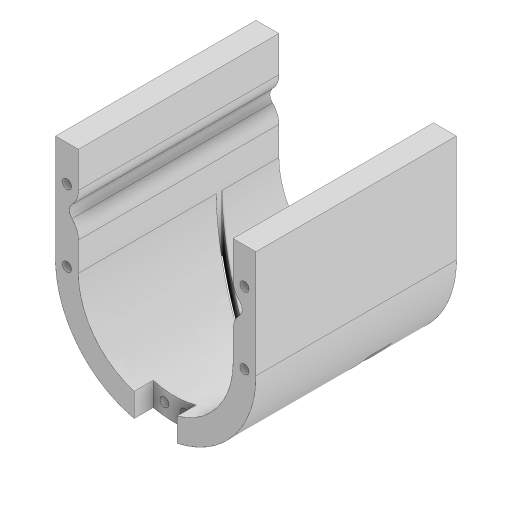
# Autodesk Inventor part: front wall
Saved by Autodesk Inventor 2024 (Build 280153000, 153)
## iProperties
Created: 2024-08-03
Part Number: front wall
Material: Generic
Document SubType Name: Modeling
Designer: chris
Density: 1 g/cm^3
Appearance: Default
Author: chris
Autodesk Inventor part; units mm, degrees
ref_plane "YZ Plane" through (0, 0, 0) normal (1, 0, 0) x (0, 1, 0)
ref_plane "XZ Plane" through (0, 0, 0) normal (0, 1, 0) x (-1, 0, 0)
ref_plane "XY Plane" through (0, 0, 0) normal (0, 0, 1) x (1, 0, 0)
sketch "Sketch1" plane through (0, 0, 0) normal (0, 0, 1) x (1, 0, 0)
  circle A0 centre (-39.37, 31.75) radius 2
  circle A1 centre (39.37, 31.75) radius 2
  circle A2 centre (39.37, 0) radius 2
  circle A3 centre (-39.37, 0) radius 2
  circle A4 centre (-4.5035, -38.773) radius 2
  circle A5 centre (4.4965, -38.773) radius 2
  arc A6 (-44.45, 0) -> (44.45, 0) centre (0, 0) ccw
  line L0 (44.45, 0) -> (44.45, 47.625)
  line L1 (-44.45, 47.625) -> (-44.45, 0)
  line L2 (-39.37, 47.625) -> (-44.45, 47.625)
  line L3 (-34.29, 37.465) -> (-34.29, 0)
  arc A7 (-34.29, 0) -> (34.29, 0) centre (0, 0) ccw
  line L4 (34.29, 0) -> (34.29, 37.465)
  line L5 (-34.29, 37.465) -> (-34.29, 47.625)
  line L6 (34.29, 37.465) -> (34.29, 47.625)
  line L7 (-39.37, 47.625) -> (-34.29, 47.625)
  line L8 (34.29, 47.625) -> (44.45, 47.625)
  circle A8 centre (198.4277, -79.2169) radius 2
  circle A9 centre (277.1677, -79.2169) radius 2
  circle A10 centre (277.1677, -110.9669) radius 2
  circle A11 centre (198.4277, -110.9669) radius 2
  circle A12 centre (233.2942, -149.74) radius 2
  circle A13 centre (242.2942, -149.74) radius 2
  arc A14 (193.3477, -110.9669) -> (282.2477, -110.9669) centre (237.7977, -110.9669) ccw
  line L9 (282.2477, -110.9669) -> (282.2477, 11.3384)
  line L10 (193.3477, 11.3384) -> (193.3477, -110.9669)
  line L11 (198.4277, -47.4669) -> (198.4277, -79.2169)
  line L12 (198.4277, -63.3419) -> (183.6023, -63.3419)
  line L13 (198.4277, -63.3419) -> (302.3131, -63.3419)
  circle A15 centre (-34.5, 22.2747) radius 2
  circle A16 centre (34.5, 22.2747) radius 2
  circle A17 centre (-34.5, 22.2747) radius 3.81
  circle A18 centre (34.5, 22.2747) radius 3.81
  point P0 (0, 0)
  point P1 (-0.0035, -24.273)
  point P2 (237.7942, -135.24)
  point P3 (-34.29, 26.0789)
  point P4 (-34.29, 18.4704)
  point P5 (34.29, 24.2636)
  point P6 (34.29, 20.2857)
  point P7 (34.29, 18.4704)
  point P8 (34.29, 26.0789)
  dimension "d8" = 7.62
  dimension "d9" = 7.62
  constraints: 28 end point, 19 centre point, 6 point on circle, 3 horizontal, 3 vertical, 2 coincident, 2 perpendicular, 1 midpoint, 2 other
  measures "d8" diameter of A17
  measures "d9" diameter of A18
extrude "Extrusion1" add sketch "Sketch1" along normal blind 88.9 contours A4 | A5 | L1 L2 L7 L5 L3 A17 A7 L4 A18 L6 L8 L0 A6 | A18 L4 A16 | L3 A15 A17 | A16 L4 | L3 A15 picked at (37.6726, 21.9824) picked at (-37.6726, 21.9824) picked at (35.4887, 22.7134) picked at (-34.6034, 21.654)
sketch "Sketch2" plane through (0, 0, 88.9) normal (0, 0, 1) x (1, 0, 0)
  arc A0 (-34.29, 0) -> (34.29, 0) centre (0, 0) ccw projected
  line L0 (0, 0) -> (0, -44.6458)
  line L1 (0, -44.6458) -> (-9.525, -44.6458)
  line L2 (-9.525, -44.6458) -> (-9.525, -25.1218)
  arc A1 (-44.45, 0) -> (44.45, 0) centre (0, 0) ccw projected
  line L3 (-44.45, 47.625) -> (-44.45, 0) projected
  arc A2 (-44.45, 0) -> (44.45, 0) centre (0, 0) ccw projected
  line L4 (44.45, 0) -> (44.45, 47.625) projected
  line L5 (44.45, 47.625) -> (34.29, 47.625) projected
  line L6 (34.29, 47.625) -> (34.29, 0) projected
  arc A3 (-34.29, 0) -> (34.29, 0) centre (0, 0) ccw projected
  line L7 (-34.29, 0) -> (-34.29, 47.625) projected
  line L8 (-34.29, 47.625) -> (-44.45, 47.625) projected
  circle A4 centre (-39.37, 31.75) radius 2 projected
  circle A5 centre (39.37, 31.75) radius 2 projected
  circle A6 centre (-39.37, 0) radius 2 projected
  circle A7 centre (39.37, 0) radius 2 projected
  line L9 (0, -44.6458) -> (9.525, -44.6458)
  line L10 (9.525, -44.6458) -> (9.525, -29.3706)
  point P0 (0, 0)
  point P1 (9.525, -43.4175)
  point P2 (9.525, -32.9405)
  point P3 (-9.525, -32.9405)
  point P4 (-9.525, -43.4175)
  dimension "d4" = 9.525
  dimension "d5" = 9.525
  constraints: 10 end point, 2 horizontal, 2 perpendicular, 1 vertical
  measures "d4" distance of L0.end L1.end
  measures "d5" distance of L0.end L9.end
extrude "Extrusion2" cut sketch "Sketch2" against normal blind 8.382 contours A0 L0 A1 L2 | A0 L10 A1 L0
extrude "Extrusion3" cut sketch "Sketch1" along normal through all contours A18 L4 A16 | L3 A15 A17 | A16 L4 | L4 A16 | L3 A15 picked at (37.6726, 21.9824) picked at (-37.6726, 21.9824) picked at (-34.6034, 21.654)
fillet "Fillet1" radius 9.525 4 edges at (34.29, 18.4704, 44.45) (34.29, 26.0789, 44.45) (-34.29, 26.0789, 44.45) (-34.29, 18.4704, 44.45)
sketch "Sketch3" plane through (-44.45, 47.625, 0) normal (0, 1, 0) x (1, 0, 0)
  line L0 (44.45, 0) -> (44.45, -92.2256)
  spline S0 degree 3 poles (23.45, -22.86) (23.45, -21.8538) (23.6516, -20.7861) (24.4574, -18.8326) (25.0612, -17.9464) (26.4629, -16.5224) (27.3659, -15.8975) (29.3494, -15.0662) (30.4304, -14.86) (32.4454, -14.86) (33.515, -15.0574) (35.4925, -15.8741) (36.4, -16.4937) (37.8226, -17.9215) (38.4359, -18.8189) (39.2496, -20.7865) (39.45, -21.8566) (39.45, -23.8634) (39.2496, -24.9335) (38.4359, -26.9011) (37.8226, -27.7985) (36.4, -29.2263) (35.4925, -29.8459) (33.515, -30.6626) (32.4454, -30.86) (30.4304, -30.86) (29.3494, -30.6538) (27.3659, -29.8225) (26.4629, -29.1976) (25.0612, -27.7736) (24.4574, -26.8874) (23.6516, -24.9339) (23.45, -23.8662) (23.45, -22.86) knots 0 0 0 0 0.301864 0.301864 0.603728 0.603728 0.917132 0.917132 1.230535 1.230535 1.536496 1.536496 1.842457 1.842457 2.143472 2.143472 2.444486 2.444486 2.7455 2.7455 3.046514 3.046514 3.352475 3.352475 3.658437 3.658437 3.97184 3.97184 4.285244 4.285244 4.587108 4.587108 4.888972 4.888972 4.888972 4.888972
  spline S1 degree 3 poles (49.45, -22.86) (49.45, -21.8566) (49.6504, -20.7865) (50.4641, -18.8189) (51.0774, -17.9215) (52.5, -16.4937) (53.4075, -15.8741) (55.385, -15.0574) (56.4546, -14.86) (58.4696, -14.86) (59.5506, -15.0662) (61.5341, -15.8975) (62.4371, -16.5224) (63.8388, -17.9464) (64.4426, -18.8326) (65.2484, -20.7861) (65.45, -21.8538) (65.45, -23.8662) (65.2484, -24.9339) (64.4426, -26.8874) (63.8388, -27.7736) (62.4371, -29.1976) (61.5341, -29.8225) (59.5506, -30.6538) (58.4696, -30.86) (56.4546, -30.86) (55.385, -30.6626) (53.4075, -29.8459) (52.5, -29.2263) (51.0774, -27.7985) (50.4641, -26.9011) (49.6504, -24.9335) (49.45, -23.8634) (49.45, -22.86) knots 0 0 0 0 0.301014 0.301014 0.602029 0.602029 0.90799 0.90799 1.213951 1.213951 1.527354 1.527354 1.840758 1.840758 2.142622 2.142622 2.444486 2.444486 2.74635 2.74635 3.048214 3.048214 3.361618 3.361618 3.675021 3.675021 3.980982 3.980982 4.286943 4.286943 4.587958 4.587958 4.888972 4.888972 4.888972 4.888972
  line L1 (10.16, -25.2412) -> (44.45, -46.2351)
  line L2 (10.16, -27.7812) -> (44.45, -48.7751)
  line L3 (78.74, -25.2412) -> (44.45, -46.2351)
  line L4 (78.74, -27.7812) -> (44.45, -48.7751)
  line L5 (44.45, 0) -> (52.6845, 8.3304)
  line L6 (10.16, 0) -> (0, 0) projected
  line L7 (0, 0) -> (0, -88.9) projected
  line L8 (10.16, -88.9) -> (0, -88.9) projected
  line L9 (10.16, 0) -> (10.16, -88.9) projected
  line L10 (88.9, 0) -> (78.74, 0) projected
  line L11 (78.74, 0) -> (78.74, -88.9) projected
  line L12 (88.9, -88.9) -> (78.74, -88.9) projected
  line L13 (88.9, 0) -> (88.9, -88.9) projected
  spline S2 degree 5 poles (24.085, -22.86) (24.0848, -22.2374) (24.1557, -21.6151) (24.2846, -21.0025) (24.6659, -19.8223) (25.2954, -18.7555) (25.6525, -18.2571) (26.4733, -17.3428) (27.4686, -16.6244) (27.9978, -16.3101) (29.113, -15.8089) (30.306, -15.5516) (30.9087, -15.476) (32.1423, -15.4643) (33.3504, -15.7079) (33.9519, -15.8877) (35.0929, -16.3878) (36.1063, -17.108) (36.5759, -17.513) (37.4191, -18.4427) (38.0595, -19.5207) (38.3264, -20.1018) (38.7089, -21.2996) (38.8487, -22.5483) (38.8487, -23.1717) (38.7089, -24.4204) (38.3264, -25.6182) (38.0595, -26.1993) (37.4191, -27.2773) (36.5759, -28.207) (36.1063, -28.612) (35.0929, -29.3322) (33.9519, -29.8323) (33.3504, -30.0121) (32.1423, -30.2557) (30.9087, -30.244) (30.306, -30.1684) (29.113, -29.9111) (27.9978, -29.4099) (27.4686, -29.0956) (26.4733, -28.3772) (25.6525, -27.4629) (25.2954, -26.9645) (24.6659, -25.8977) (24.2846, -24.7175) (24.1557, -24.1049) (24.0848, -23.4826) (24.085, -22.86) knots 0 0 0 0 0 0 0.067274 0.067274 0.067274 0.133137 0.133137 0.133137 0.199229 0.199229 0.199229 0.26442 0.26442 0.26442 0.331753 0.331753 0.331753 0.3982 0.3982 0.3982 0.466635 0.466635 0.466635 0.533365 0.533365 0.533365 0.6018 0.6018 0.6018 0.668247 0.668247 0.668247 0.73558 0.73558 0.73558 0.800771 0.800771 0.800771 0.866863 0.866863 0.866863 0.932726 0.932726 0.932726 1 1 1 1 1 1
  spline S3 degree 5 poles (50.085, -22.86) (50.0849, -22.234) (50.1564, -21.6081) (50.2867, -20.9922) (50.6747, -19.7992) (51.316, -18.7227) (51.6822, -18.2176) (52.5266, -17.2918) (53.5503, -16.5718) (54.0948, -16.257) (55.234, -15.7692) (56.4471, -15.5304) (57.0544, -15.4655) (58.2817, -15.481) (59.4794, -15.7433) (60.0689, -15.9323) (61.181, -16.4409) (62.1678, -17.1598) (62.6226, -17.5609) (63.4449, -18.4812) (64.0703, -19.5441) (64.3324, -20.1194) (64.7099, -21.3093) (64.8485, -22.5492) (64.8485, -23.1708) (64.7099, -24.4107) (64.3324, -25.6006) (64.0703, -26.1759) (63.4449, -27.2388) (62.6226, -28.1591) (62.1678, -28.5602) (61.181, -29.2791) (60.0689, -29.7877) (59.4794, -29.9767) (58.2817, -30.239) (57.0544, -30.2545) (56.4471, -30.1896) (55.234, -29.9508) (54.0948, -29.463) (53.5503, -29.1482) (52.5266, -28.4282) (51.6822, -27.5024) (51.316, -26.9973) (50.6747, -25.9208) (50.2867, -24.7278) (50.1564, -24.1119) (50.0849, -23.486) (50.085, -22.86) knots 0 0 0 0 0 0 0.06765 0.06765 0.06765 0.134655 0.134655 0.134655 0.202176 0.202176 0.202176 0.267678 0.267678 0.267678 0.334059 0.334059 0.334059 0.399058 0.399058 0.399058 0.46673 0.46673 0.46673 0.53327 0.53327 0.53327 0.600942 0.600942 0.600942 0.665941 0.665941 0.665941 0.732322 0.732322 0.732322 0.797824 0.797824 0.797824 0.865345 0.865345 0.865345 0.93235 0.93235 0.93235 1 1 1 1 1 1
  point P0 (-111.6701, 66.9173)
  point P1 (-43.0901, 66.9173)
  dimension "d27" = 0.635
  dimension "d28" = 0.635
  constraints: 12 end point, 1 vertical, 6 other
extrude "Extrusion4" cut sketch "Sketch3" against normal through all contours L3 L11 L4 L0 | L0 L2 L9 L1 | S0 | S1 | S2 | S3
chamfer "Chamfer1" distance 3.175 angle 45 6 edges at (18.9548, -40.206, 34.6302) (-18.9548, -40.206, 34.6302) (-18.9548, -40.206, 37.1702) (-34.29, -28.2842, 26.5112) (18.9548, -40.206, 37.1702) (34.29, -28.2842, 26.5112)
extrude "Extrusion5" cut sketch "Sketch1" along normal blind 12.7 contours A4 | A5
sketch "Sketch4" plane through (0, 0, 80.518) normal (0, 0, 1) x (1, 0, 0)
  circle A0 centre (4.4965, -38.773) radius 2 projected
  circle A1 centre (-4.5035, -38.773) radius 2 projected
  point P0 (0, 0)
extrude "Extrusion6" cut sketch "Sketch4" against normal blind 12.7
body "Solid1"
